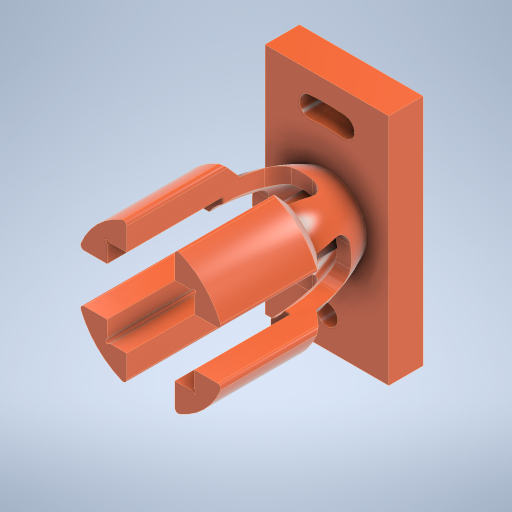
# Autodesk Inventor part: MicroRail-FlextureBase-CubeAttachment
Saved by Autodesk Inventor 2023.1 (Build 271208000, 208)
## iProperties
Created: 2023-06-05
Part Number: MicroRail-FlextureBase-CubeAttachment
Material: ABS Plastic
Document SubType Name: Modeling
Designer: hello
Density: 1.06 g/cm^3
Appearance: Smooth - Light Orange
Author: hello
Autodesk Inventor part; units mm, degrees
ref_plane "YZ Plane" through (0, 0, 0) normal (1, 0, 0) x (0, 1, 0)
ref_plane "XZ Plane" through (0, 0, 0) normal (0, 1, 0) x (-1, 0, 0)
ref_plane "XY Plane" through (0, 0, 0) normal (0, 0, 1) x (1, 0, 0)
sketch "Sketch1" plane through (0, 0, 0) normal (0, 0, 1) x (1, 0, 0)
  line L0 (-9, -17) -> (9, -17)
  line L1 (9, -17) -> (9, 17)
  line L2 (9, 17) -> (-9, 17)
  line L3 (-9, 17) -> (-9, -17)
  line L4 (-9, -17) -> (9, 17) construction
  line L5 (9, -17) -> (-9, 17) construction
  line L6 (0, -12.5) -> (0, 12.5) construction
  circle A0 centre (0, -12.5) radius 1.55
  arc A1 (2.5, 12.3747) -> (-2.5, 12.3747) centre (0, -12.5) ccw construction
  arc A2 (2.652, 13.8871) -> (-2.652, 13.8871) centre (0, -12.5) ccw
  arc A3 (2.348, 10.8623) -> (-2.348, 10.8623) centre (0, -12.5) ccw
  arc A4 (2.348, 10.8623) -> (2.652, 13.8871) centre (2.5, 12.3747) ccw
  arc A5 (-2.652, 13.8871) -> (-2.348, 10.8623) centre (-2.5, 12.3747) ccw
  point P0 (0, 0)
  dimension "d0" = 18
  dimension "d1" = 34
  dimension "d4" = 25
  dimension "d5" = 3.1
  dimension "d18" = 1.52
  dimension "d20" = 5
  constraints: 14 end point, 11 point on circle, 6 centre point, 4 tangent, 3 midpoint, 2 parallel, 1 coincident, 1 horizontal, 1 horizontal alignment, 1 perpendicular, 1 vertical, 1 vertical alignment
  measures "d0" distance of L2.end L1.end
  measures "d1" distance of L1.end L0.end
  measures "d4" distance of L6.end L6.start
  measures "d5" diameter of A0
  measures "d18" radius of A4
  measures "d20" distance of A1.end A1.start
extrude "Extrusion1" add sketch "Sketch1" along normal blind 5
sketch "Sketch6" plane through (0, 0, 5) normal (0, 0, 1) x (1, 0, 0)
  circle A0 centre (0, 0) radius 3.5
  dimension "d42" = 7
  constraints: 1 centre point, 1 coincident
  measures "d42" diameter of A0
extrude "Extrusion4" add sketch "Sketch6" along normal blind 11.65
sketch "Sketch7" plane through (0, 0, 0) normal (1, 0, 0) x (0, 1, 0)
  line L0 (-3.5, 5) -> (3.5, 5) projected
  line L1 (-17, 5) -> (17, 5) projected
  line L2 (17, 5) -> (-17, 5) projected
  line L3 (10.8623, 5) -> (10.8623, 5) projected
  line L4 (10.8623, 5) -> (13.8871, 5) projected
  line L5 (13.8871, 5) -> (13.8871, 5) projected
  line L6 (13.8871, 5) -> (10.8623, 5) projected
  line L7 (-14.05, 5) -> (-10.95, 5) projected
  line L8 (10.98, 5) -> (10.8623, 5) projected
  line L9 (0, 5) -> (0, 25.7215)
  line L10 (3.5, 16.65) -> (-3.5, 16.65) projected
  line L11 (8.5, 16.65) -> (8.5, 30.65)
  line L12 (8.5, 30.65) -> (6.5, 30.65)
  line L13 (6.5, 30.65) -> (6.5, 16.65)
  arc A0 (3.5, 5) -> (6.5, 16.65) centre (-17.6204, 16.65) ccw
  arc A1 (5.7581, 5) -> (8.5, 16.65) centre (-17.6204, 16.65) ccw
  point P0 (0, 0)
  point P1 (10.9212, 5)
  point P2 (3.5, 5)
  dimension "d47" = 17
  dimension "d49" = 14
  dimension "d67" = 2
  constraints: 8 end point, 4 point on circle, 2 centre point, 2 horizontal alignment, 2 midpoint, 2 perpendicular, 2 point on line, 2 tangent, 2 vertical, 1 concentric
  measures "d47" diameter of L11.start L9
  measures "d49" distance of L11.start L11.end
  measures "d67" distance of L11.end L12.end
revolve "Revolution2" add sketch "Sketch7" angle 360 about axis through (0, 0, 5) along (0, 0, 1)
sketch "Sketch8" plane through (0, 0, 16.65) normal (0, 0, 1) x (1, 0, 0)
  line L0 (-3.5, 10) -> (3.5, 10)
  line L1 (3.5, 10) -> (3.5, -10)
  line L2 (3.5, -10) -> (-3.5, -10)
  line L3 (-3.5, -10) -> (-3.5, 10)
  line L4 (-3.5, 10) -> (3.5, -10) construction
  line L5 (3.5, 10) -> (-3.5, -10) construction
  line L6 (-10, 3.5) -> (10, 3.5)
  line L7 (10, 3.5) -> (10, -3.5)
  line L8 (10, -3.5) -> (-10, -3.5)
  line L9 (-10, -3.5) -> (-10, 3.5)
  line L10 (-10, 3.5) -> (10, -3.5) construction
  line L11 (10, 3.5) -> (-10, -3.5) construction
  circle A0 centre (0, 0) radius 3.5 projected
  point P0 (-3.5, -3.5)
  point P1 (-3.5, 3.5)
  point P2 (3.5, -3.5)
  point P3 (3.5, 3.5)
  dimension "d52" = 20
  dimension "d53" = 20
  constraints: 24 end point, 4 midpoint, 4 parallel, 2 horizontal, 2 perpendicular, 2 tangent
  measures "d52" distance of L0.end L1.end
  measures "d53" distance of L7.end L8.end
extrude "Extrusion5" cut sketch "Sketch8" along normal blind 20 and the other way blind 8 contours L0 L1 L6 L3 | L3 L8 L9 L6 | L6 L7 L8 L1 | L8 L1 L2 L3
sketch "Sketch11" plane through (-7.746, -3.5, 30.65) normal (0, 0, 1) x (1, 0, 0)
  line L0 (4.246, -4.246) -> (4.246, -1.9772) projected
  arc A0 (2.2687, 0) -> (4.246, -1.9772) centre (7.746, 3.5) ccw projected
  line L1 (2.2687, 0) -> (0, 0) projected
  arc A1 (0, 0) -> (4.246, -4.246) centre (7.746, 3.5) ccw projected
  line L2 (0, 7) -> (2.2687, 7) projected
  arc A2 (4.246, 8.9772) -> (2.2687, 7) centre (7.746, 3.5) ccw projected
  line L3 (4.246, 8.9772) -> (4.246, 11.246) projected
  arc A3 (4.246, 11.246) -> (0, 7) centre (7.746, 3.5) ccw projected
  line L4 (13.2232, 7) -> (15.4919, 7) projected
  arc A4 (15.4919, 7) -> (11.246, 11.246) centre (7.746, 3.5) ccw projected
  line L5 (11.246, 11.246) -> (11.246, 8.9772) projected
  arc A5 (13.2232, 7) -> (11.246, 8.9772) centre (7.746, 3.5) ccw projected
  line L6 (11.246, -1.9772) -> (11.246, -4.246) projected
  arc A6 (11.246, -4.246) -> (15.4919, 0) centre (7.746, 3.5) ccw projected
  line L7 (15.4919, 0) -> (13.2232, 0) projected
  arc A7 (11.246, -1.9772) -> (13.2232, 0) centre (7.746, 3.5) ccw projected
  circle A8 centre (7.746, 3.5) radius 11
  arc A9 (0, 0) -> (4.246, -4.246) centre (7.746, 3.5) ccw projected
  line L8 (0, 0) -> (-2.6824, 0)
  line L9 (4.246, -4.246) -> (4.246, -6.9283)
  line L10 (11.246, -1.9772) -> (11.246, -4.246) projected
  line L11 (11.246, -4.246) -> (11.246, -6.9283)
  arc A10 (4.246, 11.246) -> (0, 7) centre (7.746, 3.5) ccw projected
  line L12 (0, 7) -> (-2.6824, 7)
  line L13 (4.246, 11.246) -> (4.246, 13.9283)
  line L14 (15.4919, 0) -> (18.1743, 0)
  arc A11 (15.4919, 7) -> (11.246, 11.246) centre (7.746, 3.5) ccw projected
  line L15 (11.246, 11.246) -> (11.246, 13.9283)
  line L16 (15.4919, 7) -> (18.1743, 7)
  dimension "d68" = 22
  constraints: 16 end point, 4 perpendicular, 2 horizontal, 1 coincident, 1 collinear, 1 point on line, 10 other
extrude "Extrusion7" add sketch "Sketch11" against normal up to surface (14 mm away) contours L9 A8 L8 A1 | L11 A6 L14 A8 | A8 L13 A3 L12 | A8 L16 A4 L15
chamfer "Chamfer7" distance 2.5 angle 45 4 edges at (-6.0104, 6.0104, 16.65) (-6.0104, -6.0104, 16.65) (6.0104, -6.0104, 16.65) (6.0104, 6.0104, 16.65)
sketch "Sketch12" plane through (-3.5, 5.4772, 30.65) normal (0, 0, 1) x (1, 0, 0)
  line L0 (-2.85, -11.8272) -> (9.85, -11.8272)
  line L1 (9.85, -11.8272) -> (9.85, 0.8728)
  line L2 (9.85, 0.8728) -> (-2.85, 0.8728)
  line L3 (-2.85, 0.8728) -> (-2.85, -11.8272)
  line L4 (-2.85, -11.8272) -> (9.85, 0.8728) construction
  line L5 (9.85, -11.8272) -> (-2.85, 0.8728) construction
  circle A0 centre (9.85, 0.8728) radius 0.25
  circle A1 centre (-2.85, 0.8728) radius 0.25
  circle A2 centre (-2.85, -11.8272) radius 0.25
  circle A3 centre (9.85, -11.8272) radius 0.25
  point P0 (3.5, -5.4772)
  point P1 (9.6, -11.8272)
  point P2 (9.85, -11.5772)
  point P3 (-2.85, -11.5772)
  point P4 (-2.6, -11.8272)
  point P5 (-2.6, 0.8728)
  point P6 (-2.85, 0.6228)
  point P7 (9.6, 0.8728)
  point P8 (9.85, 0.6228)
  dimension "d74" = 12.7
  dimension "d75" = 12.7
  dimension "d80" = 0.5
  dimension "d81" = 0.5
  dimension "d82" = 0.5
  dimension "d83" = 0.5
  constraints: 12 end point, 4 centre point, 4 coincident, 2 midpoint, 2 parallel, 1 horizontal, 1 perpendicular
  measures "d74" distance of L2.end L1.end
  measures "d75" distance of L1.end L0.end
  measures "d80" diameter of A0
  measures "d81" diameter of A1
  measures "d82" diameter of A2
  measures "d83" diameter of A3
extrude "Extrusion8" cut sketch "Sketch12" against normal up to surface (14 mm away)
fillet "Fillet2" radius 2 8 edges at (-5.0501, -3.5, 8.65) (5.0501, -3.5, 8.65) (-5.0501, 3.5, 8.65) (5.0501, 3.5, 8.65) (3.5, 5.0501, 8.65) (3.5, -5.0501, 8.65) (-3.5, 5.0501, 8.65) (-3.5, -5.0501, 8.65)
fillet "Fillet3" radius 0.5 8 edges at (3.5, 10.4283, 23.65) (-3.5, 10.4283, 23.65) (10.4283, 3.5, 23.65) (-10.4283, 3.5, 23.65) (-10.4283, -3.5, 23.65) (-3.5, -10.4283, 23.65) (3.5, -10.4283, 23.65) (10.4283, -3.5, 23.65)
fillet "Fillet4" radius 0.5 8 edges at (6.1, -6.35, 23.65) (6.35, -6.1, 23.65) (6.35, 6.1, 23.65) (6.1, 6.35, 23.65) (-6.1, -6.35, 23.65) (-6.35, -6.1, 23.65) (-6.35, 6.1, 23.65) (-6.1, 6.35, 23.65)
body "Solid1"
